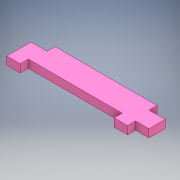
# Autodesk Inventor part: celda base cremallera
Saved by Autodesk Inventor 2018 (Build 220112000, 112)
## iProperties
Created: 2020-03-13
Part Number: celda base cremallera
Material: Genérico
Document SubType Name: Modeling
Designer: joser
Density: 1 g/cm^3
Appearance: Rosado
Author: joser
Autodesk Inventor part; units mm, degrees
ref_plane "YZ Plane" through (0, 0, 0) normal (1, 0, 0) x (0, 1, 0)
ref_plane "XZ Plane" through (0, 0, 0) normal (0, 1, 0) x (-1, 0, 0)
ref_plane "XY Plane" through (0, 0, 0) normal (0, 0, 1) x (1, 0, 0)
sketch "Boceto1" plane through (0, 0, 0) normal (0, 0, 1) x (1, 0, 0)
  line L0 (50, 0) -> (50, -6)
  line L1 (5, -9) -> (5, -6)
  line L2 (40, -6) -> (40, -9)
  line L3 (40, -9) -> (45, -9)
  line L4 (45, -9) -> (45, -6)
  line L5 (50, -6) -> (45, -6)
  line L6 (40, -6) -> (5, -6)
  line L7 (0, 0) -> (0, -9)
  line L8 (0, -9) -> (5, -9)
  line L9 (6, 0) -> (6, 3)
  line L10 (6, 3) -> (44, 3)
  line L11 (44, 3) -> (44, 0)
  line L12 (0, 0) -> (6, 0)
  line L13 (44, 0) -> (50, 0)
  dimension "d7" = 5
  dimension "d12" = 50
  dimension "d13" = 35
  dimension "d18" = 5
  dimension "d19" = 3
  dimension "d23" = 38
  dimension "d24" = 6
  dimension "d26" = 6
  dimension "d27" = 3
  constraints: 28 end point, 10 perpendicular, 5 parallel, 3 collinear, 2 horizontal, 2 vertical, 1 coincident
  measures "d7" distance of L2.end L3.end
  measures "d12" distance between parallel lines of L0 L7
  measures "d13" distance between parallel lines of L2 L1
  measures "d18" distance between parallel lines of L1 L7
  measures "d19" distance between parallel lines of L6 L8
  measures "d23" distance of L9.end L10.end
  measures "d24" distance between parallel lines of L7 L9
  measures "d26" distance between parallel lines of L5 L13
  measures "d27" distance between parallel lines of L13 L10
extrude "Extrusión1" add sketch "Boceto1" along normal blind 3
